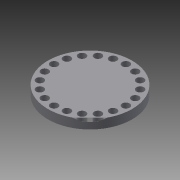
# Autodesk Inventor part: EncoderWheel2
Saved by Autodesk Inventor 2014 (Build 180170000, 170)
## iProperties
Created: 2013-05-31
Part Number: EncoderWheel2
Material: Generisch
Document SubType Name: Modeling
Designer: hanse
Density: 1 g/cm^3
Appearance: Vorgabe
Author: hanse
Autodesk Inventor part; units mm, degrees
ref_plane "YZ Plane" through (0, 0, 0) normal (1, 0, 0) x (0, 1, 0)
ref_plane "XZ Plane" through (0, 0, 0) normal (0, 1, 0) x (-1, 0, 0)
ref_plane "XY Plane" through (0, 0, 0) normal (0, 0, 1) x (1, 0, 0)
sketch "Skizze1" plane through (0, 0, 0) normal (0, 0, 1) x (1, 0, 0)
  circle A0 centre (0, 0) radius 8.4266
  circle A1 centre (0, -7.1983) radius 0.75
  circle A2 centre (2.2244, -6.846) radius 0.75
  circle A3 centre (4.2311, -5.8236) radius 0.75
  circle A4 centre (5.8236, -4.2311) radius 0.75
  circle A5 centre (6.846, -2.2244) radius 0.75
  circle A6 centre (7.1983, 0) radius 0.75
  circle A7 centre (6.846, 2.2244) radius 0.75
  circle A8 centre (5.8236, 4.2311) radius 0.75
  circle A9 centre (4.2311, 5.8236) radius 0.75
  circle A10 centre (2.2244, 6.846) radius 0.75
  circle A11 centre (0, 7.1983) radius 0.75
  circle A12 centre (-2.2244, 6.846) radius 0.75
  circle A13 centre (-4.2311, 5.8236) radius 0.75
  circle A14 centre (-5.8236, 4.2311) radius 0.75
  circle A15 centre (-6.846, 2.2244) radius 0.75
  circle A16 centre (-7.1983, 0) radius 0.75
  circle A17 centre (-6.846, -2.2244) radius 0.75
  circle A18 centre (-5.8236, -4.2311) radius 0.75
  circle A19 centre (-4.2311, -5.8236) radius 0.75
  circle A20 centre (-2.2244, -6.846) radius 0.75
  dimension "d0" = 1.5
  dimension "d3" = 360
  constraints: 21 centre point, 1 coincident, 41 other
  measures "d0" diameter of A1
extrude "Extrusion1" add sketch "Skizze1" along normal blind 1.8
